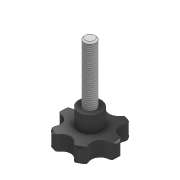
# Autodesk Inventor part: Thumb screw
Saved by Autodesk Inventor 2020 (Build 240168000, 168)
## iProperties
Created: 2022-01-21
Part Number: Thumb screw
Material: Generic
Document SubType Name: Modeling
Designer: ferrerx
Density: 1 g/cm^3
Appearance: Default
Author: ferrerx
Autodesk Inventor part; units mm, degrees
ref_plane "YZ Plane" through (0, 0, 0) normal (1, 0, 0) x (0, 1, 0)
ref_plane "XZ Plane" through (0, 0, 0) normal (0, 1, 0) x (-1, 0, 0)
ref_plane "XY Plane" through (0, 0, 0) normal (0, 0, 1) x (1, 0, 0)
sketch "Sketch1" plane through (0, 0, 0) normal (0, 1, 0) x (-1, 0, 0)
  circle A0 centre (0, 0) radius 19
  dimension "d0" = 38
  constraints: 1 centre point, 1 coincident
  measures "d0" diameter of A0
extrude "Extrusion1" add sketch "Sketch1" along normal blind 10
sketch "Sketch2" plane through (0, 10, 0) normal (0, 1, 0) x (1, 0, 0)
  circle A0 centre (0, 0) radius 7.5
  dimension "d3" = 15
  constraints: 1 centre point, 1 coincident
  measures "d3" diameter of A0
extrude "Extrusion2" add sketch "Sketch2" along normal blind 11
sketch "Sketch3" plane through (0, 21, 0) normal (0, 1, 0) x (1, 0, 0)
  circle A0 centre (0, 0) radius 4
  dimension "d6" = 8
  constraints: 1 centre point, 1 coincident
  measures "d6" diameter of A0
extrude "Extrusion3" add sketch "Sketch3" along normal blind 40
thread "Thread1" size "M8x1.25" class "6g" standard "ANSI Metric M Profile" length 180
chamfer "Chamfer1" distance 1 angle 45 1 edges at (-4, 61, 0)
chamfer "Chamfer2" distance 1 angle 45 2 edges at (19, 0, 0) (19, 10, 0)
sketch "Sketch4" plane through (0, 0, 0) normal (0, -1, 0) x (1, 0, 0)
  circle A0 centre (0, 19) radius 6
  point P0 (0, 0)
  dimension "d17" = 12
  constraints: 1 centre point
  measures "d17" diameter of A0
extrude "Extrusion4" cut sketch "Sketch4" against normal blind 40
pattern_circular "Circular Pattern1" count 6 over 360 about axis through (0, 0, 0) along (0, 1, 0) of "Extrusion4"
fillet "Fillet1" radius 3.5 12 edges at (18.5964, 5, 3.8953) (12.6717, 5, 14.1573) (5.9247, 5, 18.0526) (-5.9247, 5, 18.0526) (12.6717, 5, -14.1573) (18.5964, 5, -3.8953) (-12.6717, 5, 14.1573) (-18.5964, 5, 3.8953) (-18.5964, 5, -3.8953) (-12.6717, 5, -14.1573) (-5.9247, 5, -18.0526) (5.9247, 5, -18.0526)
body "Solid1"
